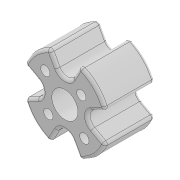
# Autodesk Inventor part: MTLV-P19
Saved by Autodesk Inventor 2020 (Build 240168000, 168)
## iProperties
Created: 2020-03-30
Part Number: MTLV-P19
Material: Generic
Document SubType Name: Modeling
Designer: John K
Density: 1 g/cm^3
Appearance: Default
Author: John K
Autodesk Inventor part; units mm, degrees
ref_plane "YZ Plane" through (0, 0, 0) normal (1, 0, 0) x (0, 1, 0)
ref_plane "XZ Plane" through (0, 0, 0) normal (0, 1, 0) x (-1, 0, 0)
ref_plane "XY Plane" through (0, 0, 0) normal (0, 0, 1) x (1, 0, 0)
sketch "Sketch1" plane through (0, 0, 0) normal (0, 0, 1) x (1, 0, 0)
  circle A0 centre (0, 0) radius 4.5
  circle A1 centre (0, 0) radius 14.75
  dimension "d0" = 9
  dimension "d1" = 29.5
  constraints: 2 centre point, 2 coincident
  measures "d0" diameter of A0
  measures "d1" diameter of A1
extrude "Extrusion1" add sketch "Sketch1" against normal mid plane 17.3
sketch "Sketch2" plane through (0, 0, 8.65) normal (0, 0, 1) x (1, 0, 0)
  line L0 (-6.7175, 6.7175) -> (6.7175, -6.7175) construction
  line L1 (-5.6569, -5.6569) -> (5.6569, 5.6569) construction
  line L2 (0, 0) -> (-8.3953, 0) construction
  dimension "d4" = 19
  dimension "d5" = 16
  dimension "d6" = 45
  constraints: 6 end point, 5 coincident, 2 midpoint, 1 horizontal, 1 perpendicular
  measures "d4" distance of L0.start L0.end
  measures "d5" distance of L1.start L1.end
  measures "d6" angle of L0 L2
hole "Hole1" at (-6.7175, 6.7175, 8.65) at (-5.6569, -5.6569, 8.65) at (6.7175, -6.7175, 8.65) at (5.6569, 5.6569, 8.65) direction (0, 0, -1) diameter 3.2 end through all clearance for "Flat Head Machine Screw" size "M3" standard "Ansi Metric M Profile"
sketch "Sketch3" plane through (0, 0, 8.65) normal (0, 0, 1) x (1, 0, 0)
  circle A0 centre (-10.75, 0) radius 3
  line L0 (-9.3117, 2.6327) -> (-13.8382, 5.1056)
  circle A1 centre (0, 0) radius 14.75 projected
  line L1 (-9.3117, -2.6327) -> (-13.8382, -5.1056)
  dimension "d14" = 6
  dimension "d15" = 10.75
  dimension "d16" = 57.296
  constraints: 4 end point, 4 point on circle, 2 tangent, 1 centre point, 1 equal length, 1 horizontal alignment
  measures "d14" diameter of A0
  measures "d15" distance of point (0, 0) A0.centre
  measures "d16" angle of L0 L1
extrude "Extrusion2" cut sketch "Sketch3" against normal through all contours A0 | A0 L1 A1 L0 picked at (-13.7366, -3.0329)
fillet "Fillet1" radius 1 2 edges at (-13.8382, 5.1056, 0) (-13.8382, -5.1056, 0)
pattern_circular "Circular Pattern1" count 4 over 360 about axis through (0, 0, 0) along (0, 0, -1) of "Fillet1", "Extrusion2"
fillet "Fillet2" radius 1 48 edges at (-11.1843, -3.6557, 8.65) (-13.5243, -5.2347, 8.65) (-10.4298, -10.4298, 8.65) (-5.2347, -13.5243, 8.65) (-3.6557, -11.1843, 8.65) (0, -7.75, 8.65) (3.6557, -11.1843, 8.65) (5.2347, -13.5243, 8.65) (10.4298, -10.4298, 8.65) (13.5243, -5.2347, 8.65) (11.1843, -3.6557, 8.65) (7.75, 0, 8.65) (11.1843, 3.6557, 8.65) (13.5243, 5.2347, 8.65) (10.4298, 10.4298, 8.65) (5.2347, 13.5243, 8.65) (3.6557, 11.1843, 8.65) (0, 7.75, 8.65) (-3.6557, 11.1843, 8.65) (-5.2347, 13.5243, 8.65) (-10.4298, 10.4298, 8.65) (-13.5243, 5.2347, 8.65) (-11.1843, 3.6557, 8.65) (-7.75, 0, 8.65) (-11.1843, 3.6557, -8.65) (-13.5243, 5.2347, -8.65) (-10.4298, 10.4298, -8.65) (-5.2347, 13.5243, -8.65) (-3.6557, 11.1843, -8.65) (0, 7.75, -8.65) (3.6557, 11.1843, -8.65) (5.2347, 13.5243, -8.65) (10.4298, 10.4298, -8.65) (13.5243, 5.2347, -8.65) (11.1843, 3.6557, -8.65) (7.75, 0, -8.65) (11.1843, -3.6557, -8.65) (13.5243, -5.2347, -8.65) (10.4298, -10.4298, -8.65) (5.2347, -13.5243, -8.65) (3.6557, -11.1843, -8.65) (0, -7.75, -8.65) (-3.6557, -11.1843, -8.65) (-5.2347, -13.5243, -8.65) (-10.4298, -10.4298, -8.65) (-13.5243, -5.2347, -8.65) (-11.1843, -3.6557, -8.65) (-7.75, 0, -8.65)
body "Solid1"
